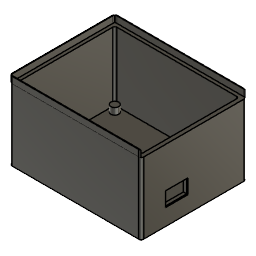
ESP32U Enclosure (Autodesk Fusion 360 design; units mm, degrees)
part number: 2026-03-11-22-37-07-836
Autodesk Fusion 360 part; units mm, degrees
sketch "Sketch1" plane through (0, 0, 0) normal (0, 0, 1) x (1, 0, 0)
  line L0 (48, 40) -> (-48, 40)
  line L1 (-50, 38) -> (-50, -38)
  line L2 (-48, -40) -> (48, -40)
  line L3 (50, -38) -> (50, 38)
  line L4 (50, 40) -> (-50, -40) construction
  line L5 (-50, 40) -> (50, -40) construction
  line L6 (45.5, 37) -> (-45.5, 37)
  line L7 (-47, 35.5) -> (-47, -35.5)
  line L8 (-45.5, -37) -> (45.5, -37)
  line L9 (47, -35.5) -> (47, 35.5)
  line L10 (47, 37) -> (-47, -37) construction
  line L11 (-47, 37) -> (47, -37) construction
  arc A0 (-48, 40) -> (-50, 38) centre (-48, 38) ccw
  arc A1 (50, 38) -> (48, 40) centre (48, 38) ccw
  arc A2 (48, -40) -> (50, -38) centre (48, -38) ccw
  arc A3 (-50, -38) -> (-48, -40) centre (-48, -38) ccw
  arc A4 (-45.5, 37) -> (-47, 35.5) centre (-45.5, 35.5) ccw
  arc A5 (47, 35.5) -> (45.5, 37) centre (45.5, 35.5) ccw
  arc A6 (45.5, -37) -> (47, -35.5) centre (45.5, -35.5) ccw
  arc A7 (-47, -35.5) -> (-45.5, -37) centre (-45.5, -35.5) ccw
  dimension "d1" = 100
  dimension "d2" = 80
  dimension "d3" = 94
  dimension "d4" = 74
  dimension "d5" = 2
  dimension "d6" = 1.5
  constraint horizontal L0
  constraint perpendicular L0 L1
  constraint parallel L0 L2
  constraint parallel L1 L3
  constraint coincident L4 origin
  constraint coincident L5 origin
  constraint horizontal L6
  constraint perpendicular L6 L7
  constraint parallel L6 L8
  constraint parallel L7 L9
  constraint coincident L10 origin
  constraint coincident L11 origin
  constraint coincident L5.start L1
  constraint coincident L5.start L0
  constraint tangent L1 A0
  constraint tangent L0 A0
  constraint coincident L4.start L0
  constraint coincident L4.start L3
  constraint tangent L0 A1
  constraint tangent L3 A1
  constraint equal A0 A1
  constraint coincident L5.end L3
  constraint coincident L5.end L2
  constraint tangent L3 A2
  constraint tangent L2 A2
  constraint equal A0 A2
  constraint coincident L4.end L2
  constraint coincident L4.end L1
  constraint tangent L2 A3
  constraint tangent L1 A3
  constraint equal A0 A3
  constraint coincident L11.start L7
  constraint coincident L11.start L6
  constraint tangent L7 A4
  constraint tangent L6 A4
  constraint coincident L10.start L6
  constraint coincident L10.start L9
  constraint tangent L6 A5
  constraint tangent L9 A5
  constraint equal A4 A5
  constraint coincident L11.end L9
  constraint coincident L11.end L8
  constraint tangent L9 A6
  constraint tangent L8 A6
  constraint equal A4 A6
  constraint coincident L10.end L8
  constraint coincident L10.end L7
  constraint tangent L8 A7
  constraint tangent L7 A7
  constraint equal A4 A7
  measures "d1" distance of L4.end L5.end
  measures "d2" distance of L5.start L4.end
  measures "d3" distance of L10.end L11.end
  measures "d4" distance of L11.start L10.end
  measures "d5" radius of A0
  measures "d6" radius of A4
extrude "Extrude1" add sketch "Sketch1" along normal blind 55
extrude "Extrude2" add sketch "Sketch1" along normal blind 3 contours L6 L7 L8 L9 A4 A5 A6 A7
chamfer "Chamfer1" distance 1 angle 45 8 edges at (50, 0, 0) (49.4142, 39.4142, 0) (0, 40, 0) (-49.4142, 39.4142, 0) (-50, 0, 0) (-49.4142, -39.4142, 0) (0, -40, 0) (49.4142, -39.4142, 0)
sketch "Sketch2" plane through (0, 0, 3) normal (0, 0, 1) x (-1, 0, 0)
  arc A0 (47, 35.5) -> (45.5, 37) centre (45.5, 35.5) ccw
  line L0 (45.5, 37) -> (-45.5, 37)
  arc A1 (-45.5, 37) -> (-47, 35.5) centre (-45.5, 35.5) ccw
  line L1 (-47, 35.5) -> (-47, -35.5)
  arc A2 (-47, -35.5) -> (-45.5, -37) centre (-45.5, -35.5) ccw
  line L2 (-45.5, -37) -> (45.5, -37)
  arc A3 (45.5, -37) -> (47, -35.5) centre (45.5, -35.5) ccw
  line L3 (47, -35.5) -> (47, 35.5)
  circle A4 centre (42.5, -32.5) radius 3
  line L4 (50, 0) -> (-50, 0) construction
  line L5 (0, -40) -> (0, 40) construction
  circle A5 centre (42.5, 32.5) radius 3
  circle A6 centre (-42.5, -32.5) radius 3
  circle A7 centre (-42.5, 32.5) radius 3
  dimension "d12" = 6
  dimension "d13" = 4.5
  dimension "d14" = 4.5
  constraint perpendicular L1 L4
  constraint perpendicular L0 L5
  constraint symmetric A4 L4 A5
  constraint symmetric A4 L5 A6
  constraint symmetric L5 A5 A7
  measures "d12" diameter of A4
  measures "d13" distance of L2 A4.centre
  measures "d14" distance of L3 A4.centre
extrude "Extrude3" add sketch "Sketch2" along normal blind 5 contours A4 | A5 | A6 | A7
sketch "Sketch3" plane through (50, 0, 0) normal (1, 0, 0) x (0, 1, 0)
  line L0 (-38, 1) -> (38, 1)
  line L1 (38, 1) -> (38, 55)
  line L2 (38, 55) -> (-38, 55)
  line L3 (-38, 55) -> (-38, 1)
  line L4 (-5, 24) -> (-21, 24)
  line L5 (-21, 24) -> (-21, 14)
  line L6 (-21, 14) -> (-5, 14)
  line L7 (-5, 14) -> (-5, 24)
  line L8 (-5, 24) -> (-21, 14) construction
  line L9 (-21, 24) -> (-5, 14) construction
  point P0 (-13, 19)
  dimension "d17" = 16
  dimension "d18" = 10
  dimension "d19" = 25
  dimension "d20" = 18
  constraint horizontal L4
  constraint perpendicular L4 L5
  constraint parallel L4 L6
  constraint parallel L5 L7
  constraint coincident L8 P0
  constraint coincident L9 P0
  measures "d17" distance of L5.end L6.end
  measures "d18" distance of L4.end L5.end
  measures "d19" distance of L3 P0
  measures "d20" distance of L0 P0
extrude "Extrude4" cut sketch "Sketch3" against normal blind 3 contours L4 L5 L6 L7
sketch "Sketch4" plane through (0, 40, 0) normal (0, 1, 0) x (-1, 0, 0)
  line L0 (-48, 1) -> (48, 1)
  line L1 (48, 1) -> (48, 55)
  line L2 (48, 55) -> (-48, 55)
  line L3 (-48, 55) -> (-48, 1)
  circle A0 centre (-36, 31) radius 3.5
  dimension "d23" = 7
  dimension "d24" = 12
  dimension "d25" = 30
  measures "d23" diameter of A0
  measures "d24" distance of L3 A0.centre
  measures "d25" distance of L0 A0.centre
extrude "Extrude5" cut sketch "Sketch4" against normal blind 3 contours A0
extrude "Extrude6" add 1 faces at (-15.1667, 39, 55) along direction (0, 0, 1) blind 5
sketch "Sketch5" plane through (0, 0, 60) normal (0, 0, 1) x (-1, 0, 0)
  arc A0 (47, 35.5) -> (45.5, 37) centre (45.5, 35.5) ccw
  line L0 (47, 35.5) -> (47, -35.5)
  arc A1 (45.5, -37) -> (47, -35.5) centre (45.5, -35.5) ccw
  line L1 (45.5, -37) -> (-45.5, -37)
  arc A2 (-47, -35.5) -> (-45.5, -37) centre (-45.5, -35.5) ccw
  line L2 (-47, -35.5) -> (-47, 35.5)
  arc A3 (-45.5, 37) -> (-47, 35.5) centre (-45.5, 35.5) ccw
  line L3 (-45.5, 37) -> (45.5, 37)
  arc A4 (50, 38) -> (48, 40) centre (48, 38) ccw
  line L4 (48, 40) -> (-48, 40)
  arc A5 (-48, 40) -> (-50, 38) centre (-48, 38) ccw
  line L5 (-50, 38) -> (-50, -38)
  arc A6 (-50, -38) -> (-48, -40) centre (-48, -38) ccw
  line L6 (-48, -40) -> (48, -40)
  arc A7 (48, -40) -> (50, -38) centre (48, -38) ccw
  line L7 (50, -38) -> (50, 38)
  line L8 (49.5, 39.5) -> (-49.5, 39.5)
  line L9 (-49.5, 39.5) -> (-49.5, -39.5)
  line L10 (-49.5, -39.5) -> (49.5, -39.5)
  line L11 (49.5, -39.5) -> (49.5, 39.5)
  line L12 (46.3, 36.3) -> (-46.3, 36.3)
  line L13 (-46.3, 36.3) -> (-46.3, -36.3)
  line L14 (-46.3, -36.3) -> (46.3, -36.3)
  line L15 (46.3, -36.3) -> (46.3, 36.3)
  dimension "d30" = 0.5
  dimension "d31" = 0.5
  dimension "d32" = 0.5
  dimension "d33" = 0.5
  dimension "d34" = 3.2
  dimension "d35" = 3.2
  dimension "d36" = 3.2
  dimension "d37" = 3.2
  measures "d30" distance of L7 L11
  measures "d31" distance of L4 L8
  measures "d32" distance of L6 L10
  measures "d33" distance of L5 L9
  measures "d34" distance of L8 L12
  measures "d35" distance of L11 L15
  measures "d36" distance of L10 L14
  measures "d37" distance of L9 L13
extrude "Extrude7" cut sketch "Sketch5" against normal blind 5 contours A0 L0 A1 L1 A2 L2 A3 L3 | A4 A5 A6 A7 L8 L9 L10 L11
extrude "Extrude8" cut 1 faces at (49.6667, 12.6667, 60) along direction (0, 0, -1) blind 5
chamfer "Chamfer2" distance 0.5 angle 45 4 edges at (50, -5, 19) (50, -13, 24) (50, -21, 19) (50, -13, 14)
chamfer "Chamfer3" distance 0.5 angle 45 1 edges at (39.2631, 40, 32.2657)
